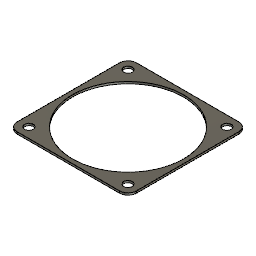
Zentralstecker_Motor_W461 (Autodesk Fusion 360 design; units mm, degrees)
part number: 2026-04-15-17-27-10-843
Autodesk Fusion 360 part; units mm, degrees
sketch "Sketch1" plane through (0, 0, 0) normal (0, 0, 1) x (1, 0, 0)
  line L0 (30, -35) -> (-30, -35)
  line L1 (-35, -30) -> (-35, 30)
  line L2 (-30, 35) -> (30, 35)
  line L3 (35, 30) -> (35, -30)
  line L4 (35, -35) -> (-35, 35) construction
  line L5 (-35, -35) -> (35, 35) construction
  circle A0 centre (0, 0) radius 32.5
  circle A1 centre (-28.9896, 28.9896) radius 2.5
  arc A2 (-30, 35) -> (-35, 30) centre (-30, 30) ccw
  arc A3 (35, 30) -> (30, 35) centre (30, 30) ccw
  arc A4 (30, -35) -> (35, -30) centre (30, -30) ccw
  arc A5 (-35, -30) -> (-30, -35) centre (-30, -30) ccw
  line L6 (0, 35) -> (0, -35) construction
  line L7 (-35, 0) -> (35, 0) construction
  circle A6 centre (28.9896, 28.9896) radius 2.5
  circle A7 centre (-28.9896, -28.9896) radius 2.5
  circle A8 centre (28.9896, -28.9896) radius 2.5
  dimension "d1" = 70
  dimension "d2" = 70
  dimension "d3" = 65
  dimension "d4" = 5
  dimension "d5" = 8.5
  dimension "d6" = 5
  dimension "d7" = 5
  dimension "d8" = 5
  dimension "d9" = 5
  constraint horizontal L0
  constraint perpendicular L0 L1
  constraint parallel L0 L2
  constraint parallel L1 L3
  constraint coincident L4 A0.centre
  constraint coincident L5 A0.centre
  constraint coincident A0.centre origin
  constraint coincident L4 A1.centre
  constraint coincident L4.end L1
  constraint coincident L4.end L2
  constraint tangent L1 A2
  constraint tangent L2 A2
  constraint coincident L5.end L2
  constraint coincident L5.end L3
  constraint tangent L2 A3
  constraint tangent L3 A3
  constraint coincident L4.start L3
  constraint coincident L4.start L0
  constraint tangent L3 A4
  constraint tangent L0 A4
  constraint coincident L5.start L0
  constraint coincident L5.start L1
  constraint tangent L0 A5
  constraint tangent L1 A5
  constraint midpoint L2 L6.start
  constraint midpoint L0 L6.end
  constraint midpoint L1 L7.start
  constraint perpendicular L6 L7
  constraint symmetric A1 L6 A6
  constraint symmetric A1 L7 A7
  constraint symmetric L7 A6 A8
  measures "d1" distance of L4.end L5.end
  measures "d2" distance of L5.start L4.end
  measures "d3" diameter of A0
  measures "d4" diameter of A1
  measures "d5" distance of L4.end A1.centre
  measures "d6" radius of A2
  measures "d7" radius of A3
  measures "d8" radius of A4
  measures "d9" radius of A5
extrude "Extrude1" add sketch "Sketch1" along normal blind 1.2
